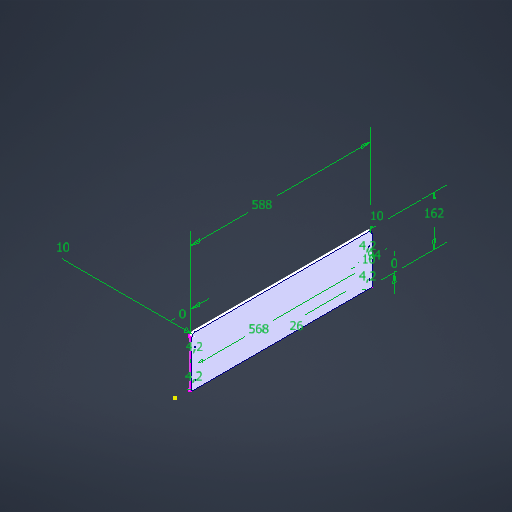
# Autodesk Inventor part: Plexiglasabdeckung
Saved by Autodesk Inventor 2026.1 (Build 301233020, 233B)
## iProperties
Created: 2026-03-07
Part Number: Plexiglasabdeckung
Material: Polycarbonat, rauchfarben
Document SubType Name: Modeling
Designer: neume
Density: 1.2 g/cm^3
Appearance: Polycarbonat - Rauch
Source: unknown
Author: neume
Autodesk Inventor part; units mm, degrees
ref_plane "YZ Plane" through (0, 0, 0) normal (1, 0, 0) x (0, 1, 0)
ref_plane "XZ Plane" through (0, 0, 0) normal (0, 1, 0) x (-1, 0, 0)
ref_plane "XY Plane" through (0, 0, 0) normal (0, 0, 1) x (1, 0, 0)
sketch "Skizze1" plane through (0, 0, 0) normal (1, 0, 0) x (0, 1, 0)
  line L0 (149, -51) -> (-3, -51)
  line L1 (-3, -51) -> (-3, -639)
  line L2 (-3, -639) -> (149, -639)
  line L3 (159, -629) -> (159, -61)
  arc A0 (159, -61) -> (149, -51) centre (149, -61) ccw
  line L4 (-3, -51) -> (149, -51) projected
  line L5 (-3, -51) -> (-3, -639) projected
  arc A1 (149, -639) -> (159, -629) centre (149, -629) ccw
  line L6 (117, -61) -> (23, -61) construction
  line L7 (23, -61) -> (23, -629) construction
  line L8 (23, -629) -> (117, -629) construction
  line L9 (117, -629) -> (117, -61) construction
  circle A2 centre (117, -61) radius 2.1
  circle A3 centre (117, -629) radius 2.1
  circle A4 centre (23, -629) radius 2.1
  circle A5 centre (23, -61) radius 2.1
  point P0 (0, 0)
  point P1 (73, -639)
  dimension "d0" = 10
  dimension "d3" = 588
  dimension "d4" = 162
  dimension "d5" = 0
  dimension "d6" = 0
  dimension "d7" = 10
  dimension "d8" = 4.2
  dimension "d9" = 4.2
  dimension "d10" = 4.2
  dimension "d11" = 4.2
  dimension "d12" = 568
  dimension "d13" = 94
  dimension "d14" = 26
  dimension "d15" = 10
  constraints: 16 end point, 6 centre point, 4 coincident, 4 parallel, 4 point on circle, 4 tangent, 2 horizontal, 2 perpendicular, 1 midpoint
  measures "d0" radius of A0
  measures "d3" distance from line of point (73, -639) L0
  measures "d4" distance between parallel lines of L3 L1
  measures "d5" distance between parallel lines of L4 L0
  measures "d6" distance between parallel lines of L5 L1
  measures "d7" radius of A1
  measures "d8" diameter of A2
  measures "d9" diameter of A5
  measures "d10" diameter of A4
  measures "d11" diameter of A3
  measures "d12" distance between parallel lines of L6 L8
  measures "d13" distance between parallel lines of L9 L7
  measures "d14" distance between parallel lines of L1 L7
  measures "d15" distance between parallel lines of L2 L8
extrude "Extrusion1" add sketch "Skizze1" along normal blind 5 contours A0 L3 A1 L2 L1 L0 | A2 | A3 | A4 | A5
extrude "Extrusion2" cut sketch "Skizze1" along normal blind 5 contours A2 | A3 | A4 | A5
